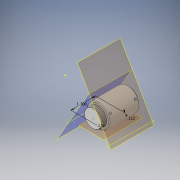
# Autodesk Inventor part: laserfocus
Saved by Autodesk Inventor 2019 (Build 230136000, 136)
## iProperties
Created: 2019-03-07
Part Number: laserfocus
Material: Generic
Document SubType Name: Modeling
Designer: Saumya
Density: 1 g/cm^3
Appearance: Default
Author: Saumya
Autodesk Inventor part; units mm, degrees
ref_plane "YZ Plane" through (0, 0, 0) normal (1, 0, 0) x (0, 1, 0)
ref_plane "XY Plane" through (0, 0, 0) normal (0, 0, 1) x (1, 0, 0)
sketch "Sketch1" plane through (0, 0, 0) normal (0, 0, 1) x (1, 0, 0)
  circle A0 centre (84.114, 58.3351) radius 15.24
  line L0 (84.114, 61.4651) -> (84.114, 53.9668)
  line L1 (87.092, 58.3351) -> (81.5348, 58.3351)
  point P0 (0, 0)
  dimension "d0" = 30.48
  constraints: 4 end point, 1 centre point, 1 horizontal, 1 vertical
  measures "d0" diameter of A0
extrude "Extrusion1" add sketch "Sketch1" along normal blind 40.64
sketch "Sketch2" plane through (84.114, 58.3351, 40.64) normal (0, 0, 1) x (1, 0, 0)
  circle A0 centre (0, 0) radius 11.8999
  circle A1 centre (0, 0) radius 0.381
  point P0 (-84.114, -58.3351)
  dimension "d3" = 23.7998
  dimension "d62" = 0.762
  constraints: 2 centre point, 1 coincident
  measures "d3" diameter of A0
  measures "d62" diameter of A1
extrude "Extrusion2" add sketch "Sketch2" along normal blind 6.35 contours A0 | A1
chamfer "Chamfer1" distance 0.508 angle 45 1 edges at (72.2141, 58.3351, 46.99)
chamfer "Chamfer2" distance 1.016 angle 45 1 edges at (68.874, 58.3351, 40.64)
thread "Thread2" size "M25x1" class "6g" standard "ANSI Metric M Profile" full length
sketch "Sketch4" plane through (84.114, 58.3351, 0) normal (0, 0, -1) x (-1, 0, 0)
  circle A0 centre (0, 0) radius 11.8999 projected
  point P0 (84.114, -58.3351)
  constraints: 1 coincident
hole "Hole1" at (84.114, 58.3351, 0) direction (0, 0, 1) diameter 15.24 depth 41.91 tip angle 120
chamfer "Chamfer3" distance 1.016 angle 45 1 edges at (68.874, 58.3351, 0)
sketch "Sketch9" plane through (84.114, 58.3351, 46.99) normal (0, 0, 1) x (1, 0, 0)
  point P0 (0, 0)
hole "Hole3" at (84.114, 58.3351, 46.99) direction (0, 0, 1) diameter 0.762 depth 41.91 tip angle 120
sketch "Sketch10" plane through (84.114, 58.3351, 46.99) normal (0, 0, 1) x (1, 0, 0)
  circle A0 centre (0, 0) radius 0.381
  point P0 (-84.114, -58.3351)
  dimension "d63" = 0.762
  constraints: 1 centre point
  measures "d63" diameter of A0
extrude "Extrusion6" cut sketch "Sketch10" against normal blind 7.62
ref_plane "Work Plane11" through (84.114, 43.0951, 0) normal (0, 1, 0) x (-1, 0, 0)
sketch "Sketch12" plane through (84.114, 43.0951, 0) normal (0, 1, 0) x (-1, 0, 0)
  circle A0 centre (0, 36.83) radius 1.4224
  circle A1 centre (0, 3.81) radius 1.4224
  point P0 (84.114, 0)
  dimension "d68" = 2.8448
  dimension "d69" = 2.8448
  dimension "d71" = 33.02
  constraints: 2 centre point
  measures "d68" diameter of A0
  measures "d69" diameter of A1
  measures "d71" distance of A0.centre A1.centre
sketch "Sketch19" plane through (84.114, 43.0951, 0) normal (0, 1, 0) x (-1, 0, 0)
  point P0 (84.114, 0)
sketch "Sketch20" plane through (84.114, 43.0951, 0) normal (0, 1, 0) x (-1, 0, 0)
  circle A0 centre (-0.009, 36.83) radius 1.27
  circle A1 centre (-0.009, 3.81) radius 1.27
  line L0 (-11.3919, 46.99) -> (11.3919, 46.99) projected
  point P0 (84.114, 0)
  dimension "d78" = 2.54
  dimension "d79" = 2.54
  dimension "d80" = 10.16
  dimension "d81" = 33.02
  constraints: 2 centre point
  measures "d78" diameter of A0
  measures "d79" diameter of A1
  measures "d80" distance from line of A0.centre L0
  measures "d81" distance of A0.centre A1.centre
extrude "Extrusion9" cut sketch "Sketch20" along normal blind 8.89
sketch "Sketch21" plane through (84.114, 43.0951, 0) normal (0, 1, 0) x (-1, 0, 0)
  point P0 (84.114, 0)
sketch "Sketch22" plane through (84.114, 43.0951, 0) normal (0, 1, 0) x (-1, 0, 0)
  point P0 (84.114, 0)
  point P1 (27.3328, 48.7683)
  point P2 (26.9749, -2.1467)
  point P3 (-27.3472, -1.8634)
  point P4 (-26.971, 48.9999)
ref_plane "Work Plane17" through (57.1391, 43.0951, -2.1467) normal (-0.866, 0.5, -0.0061) x (-0.007, 0, 1)
sketch "Sketch23" plane through (57.1391, 43.0951, -2.1467) normal (-0.866, 0.5, -0.0061) x (-0.007, 0, 1)
  circle A0 centre (38.7859, 26.8321) radius 1.4224
  circle A1 centre (5.7659, 26.8321) radius 1.4224
  ellipse E0 centre (48.9459, 26.858) end of major axis (48.9058, 38.2499) minor radius 0.0694 projected
  point P0 (2.5484, -65.8828)
  dimension "d88" = 2.8448
  dimension "d89" = 2.8448
  dimension "d90" = 10.16
  dimension "d91" = 33.02
  constraints: 2 centre point, 1 other
  measures "d88" diameter of A0
  measures "d89" diameter of A1
  measures "d90" horizontal distance of A0.centre point (48.946, 26.858)
  measures "d91" distance of A1.centre A0.centre
extrude "Extrusion10" cut sketch "Sketch23" against normal blind 8.89 contours A0 | A1
ref_plane "Work Plane18" through (111.085, 43.0951, 48.9999) normal (0.866, 0.5, 0.0064) x (0.0074, 0, -1)
sketch "Sketch24" plane through (111.085, 43.0951, 48.9999) normal (0.866, 0.5, 0.0064) x (0.0074, 0, -1)
  circle A0 centre (11.9704, 26.7143) radius 1.4224
  circle A1 centre (44.9904, 26.7143) radius 1.4224
  ellipse E0 centre (1.8104, 26.6908) end of major axis (1.7683, 38.0826) minor radius 0.073 projected
  point P0 (48.177, 18.4007)
  dimension "d95" = 2.8448
  dimension "d96" = 2.8448
  dimension "d97" = 10.16
  dimension "d98" = 33.02
  constraints: 2 centre point, 1 other
  measures "d95" diameter of A0
  measures "d96" diameter of A1
  measures "d97" horizontal distance of A0.centre point (1.81, 26.691)
  measures "d98" distance of A1.centre A0.centre
extrude "Extrusion11" cut sketch "Sketch24" against normal blind 8.89 contours A0 | A1
thread "Thread3" size "4-40 UNC" class "2B" standard "ANSI Unified Screw Threads" full length
body "Solid1"
